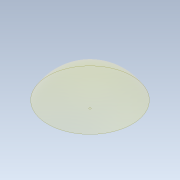
# Autodesk Inventor part: lens_FoV
Saved by Autodesk Inventor 2020 (Build 240168000, 168)
## iProperties
Created: 2021-02-15
Part Number: lens_FoV
Material: Generic
Document SubType Name: Modeling
Designer: DELL
Density: 1 g/cm^3
Appearance: Default
Author: DELL
Autodesk Inventor part; units mm, degrees
ref_plane "YZ Plane" through (0, 0, 0) normal (1, 0, 0) x (0, 1, 0)
ref_plane "XZ Plane" through (0, 0, 0) normal (0, 1, 0) x (-1, 0, 0)
ref_plane "XY Plane" through (0, 0, 0) normal (0, 0, 1) x (1, 0, 0)
sketch "Sketch1" plane through (0, 0, 0) normal (0, 0, 1) x (1, 0, 0)
  line L0 (-5.5, 0) -> (5.5, 0)
  line L1 (5.5, 0) -> (262.4601, 45.309)
  line L2 (0, 0) -> (0, 200) construction
  line L3 (-5.5, 0) -> (-262.4601, 45.309)
  arc A0 (262.4601, 45.309) -> (-262.4601, 45.309) centre (0, -100) ccw
  line L4 (0, 0) -> (0, 200)
  dimension "d0" = 80
  dimension "d1" = 11
  dimension "d2" = 200
  dimension "d3" = 600
  constraints: 10 end point, 3 point on circle, 2 vertical, 1 centre point, 1 coincident, 1 horizontal, 1 midpoint, 1 point on line, 1 symmetric about line
  measures "d0" angle of L2 L1
  measures "d1" distance of L0.start L0.end
  measures "d2" distance of L2.start L2.end
  measures "d3" diameter of A0
revolve "Revolution1" add sketch "Sketch1" angle 360 about axis through (0, 0, 0) along (0, 1, 0) contours L3 A0 L4 L0
body "Solid1"
